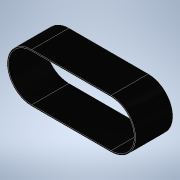
# Autodesk Inventor part: Polyurethane Belt STOCK
Saved by Autodesk Inventor 2022 (Build 260153000, 153)
## iProperties
Created: 2020-01-25
Part Number: Polyurethane Belt STOCK
Material: Rubber
Document SubType Name: Modeling
Designer: aidan
Density: 0.93 g/cm^3
Appearance: Anodized - Black
Author: aidan
Autodesk Inventor part; units mm, degrees
ref_plane "YZ Plane" through (0, 0, 0) normal (1, 0, 0) x (0, 1, 0)
ref_plane "XZ Plane" through (0, 0, 0) normal (0, 1, 0) x (-1, 0, 0)
ref_plane "XY Plane" through (0, 0, 0) normal (0, 0, 1) x (1, 0, 0)
sketch "Sketch1" plane through (0, 0, 0) normal (0, 0, 1) x (1, 0, 0)
  arc A0 (-13.4919, 42.7251) -> (-13.4919, -20.7749) centre (-13.4919, 10.9751) ccw
  arc A1 (94.4581, -20.7749) -> (94.4581, 42.7251) centre (94.4581, 10.9751) ccw
  line L0 (-13.4919, 42.7251) -> (94.4581, 42.7251)
  line L1 (94.4581, -20.7749) -> (-13.4919, -20.7749)
  line L2 (94.4581, 44.3126) -> (-13.4919, 44.3126)
  arc A2 (-13.4919, 44.3126) -> (-13.4919, -22.3624) centre (-13.4919, 10.9751) ccw
  line L3 (-13.4919, -22.3624) -> (94.4581, -22.3624)
  arc A3 (94.4581, -22.3624) -> (94.4581, 44.3126) centre (94.4581, 10.9751) ccw
  point P0 (0, 0)
  dimension "d2" = 31.75
  dimension "d3" = 107.95
  dimension "d4" = 1.5875
  constraints: 8 end point, 8 point on circle, 4 centre point, 3 tangent, 2 parallel, 1 equal radius, 1 horizontal, 3 other
  measures "d2" radius of A0
  measures "d3" distance of L0.start L0.end
  measures "d4" distance between parallel lines of L0 L2
extrude "Extrusion1" add sketch "Sketch1" along normal blind 50.8
equation "\"d2\" = d1"
equation "\"d3\" = d0"
equation "\"d0\" = 107.95"
equation "\"d1\" = 31.75"
body "Solid1"
